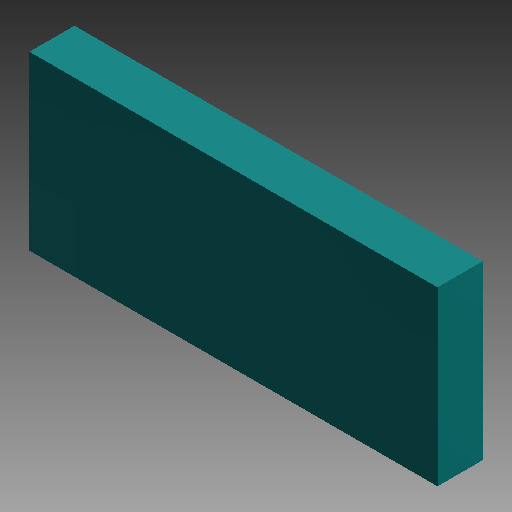
# Autodesk Inventor part: Header 5X2
Saved by Autodesk Inventor 2018.2 (Build 222227000, 227)
## iProperties
Part Number: Header 5X2
Material: Generic
Document SubType Name: Modeling
Designer: autocad
Appearance: HDR2X5, Header 5X2
Author: autocad
Autodesk Inventor part; units mm, degrees
ref_plane "YZ Plane" through (0, 0, 0) normal (1, 0, 0) x (0, 1, 0)
ref_plane "XZ Plane" through (0, 0, 0) normal (0, 1, 0) x (-1, 0, 0)
ref_plane "XY Plane" through (0, 0, 0) normal (0, 0, 1) x (1, 0, 0)
sketch "HDR2X5, Header 5X2_8" plane through (0, 0, 0) normal (0, 0, 1) x (1, 0, 0)
  line L0 (-2.7246, -3.3525) -> (14.479, -3.3525)
  line L1 (14.479, -3.3525) -> (14.479, 3.91)
  line L2 (14.479, 3.91) -> (-2.7246, 3.91)
  line L3 (-2.7246, 3.91) -> (-2.7246, -3.3525)
  constraints: 8 end point
extrude "Extrusion1" add sketch "HDR2X5, Header 5X2_8" along normal blind 1.9
body "Solid1"
